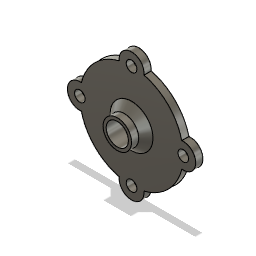
Diode_Holder_Mirror_Mount v5 (Autodesk Fusion 360 design; units mm, degrees)
Autodesk Fusion 360 part; units mm, degrees
note: some values were not read from the file. Set by a fixed rule: which sketch regions a step uses.
sketch "Sketch1" plane through (0, 0, 0) normal (0, 0, 1) x (1, 0, 0)
  circle A0 centre (0, 0) radius 11
  circle A1 centre (0, 0) radius 12.5
  circle A2 centre (0, 0) radius 14.5
  line L0 (0, 0) -> (0, 14.5)
  line L1 (0, 0) -> (14.5, 0)
  line L2 (0, 0) -> (-14.5, 0)
  line L3 (0, 0) -> (0, -14.5)
  circle A3 centre (0, 14.5) radius 3.5
  circle A4 centre (14.5, 0) radius 3.5
  circle A5 centre (0, -14.5) radius 3.5
  circle A6 centre (-14.5, 0) radius 3.5
  circle A7 centre (-14.5, 0) radius 1.5
  circle A8 centre (0, 14.5) radius 1.5
  circle A9 centre (14.5, 0) radius 1.5
  circle A10 centre (0, -14.5) radius 1.5
  dimension "d1" = 22
  dimension "d2" = 25
  dimension "d3" = 29
  dimension "d4" = 7
  dimension "d5" = 3
  dimension "d6" = 3
  dimension "d7" = 3
  dimension "d8" = 3
  constraint coincident A0.centre A1.centre
  constraint coincident A2 L0.end
  constraint vertical L0
  constraint coincident A2 L1.end
  constraint perpendicular L0 L1
  constraint coincident A2 L2.end
  constraint perpendicular L0 L2
  constraint coincident A2 L3.end
  constraint perpendicular L2 L3
  constraint coincident L0.end A3.centre
  constraint coincident L1.end A4.centre
  constraint tangent A0 A4
  constraint coincident L3.end A5.centre
  constraint tangent A0 A5
  constraint coincident L2.end A6.centre
  constraint concentric A6 A7
  constraint concentric A3 A8
  constraint concentric A4 A9
  constraint concentric A5 A10
  measures "d1" diameter of A0
  measures "d2" diameter of A1
  measures "d3" diameter of A2
  measures "d4" diameter of A3
  measures "d5" diameter of A7
  measures "d6" diameter of A8
  measures "d7" diameter of A9
  measures "d8" diameter of A10
extrude "Extrude1" add sketch "Sketch1" along normal blind 1 contours A0 A1 A4 A5 | A1 L1 A4 | A0 A1 A3 A4 | A1 L1 A4 | A1 L0 A3 | A0 A1 A3 A6 | A1 L0 A3 | A0 A1 A5 A6 | A1 L3 A5 | A1 L3 A5 | A1 A2 L1 A4 A9 | A1 A2 L1 A4 A9 | A1 A2 A3 A4 | A1 A2 A4 A5 | A1 L2 A6 | A1 L2 A6 | A1 A2 L0 A3 A8 | A1 A2 L0 A3 A8 | A1 A2 A3 A6 | A1 A2 L3 A5 A10 | A1 A2 L3 A5 A10 | A1 A2 A5 A6 | A2 A4 A9 | A1 A2 L2 A6 A7 | A1 A2 L2 A6 A7 | A2 A3 A8 | A2 A5 A10 | A2 A6 A7
sketch "Sketch2" plane through (0, 0, 1) normal (0, 0, 1) x (1, 0, 0)
  circle A0 centre (0, -14.5) radius 1.5
  circle A1 centre (14.5, 0) radius 1.5
  circle A2 centre (-14.5, 0) radius 1.5
  circle A3 centre (0, 14.5) radius 1.5
  circle A4 centre (0, 0) radius 11
  arc A5 (-3.4744, 14.0776) -> (-14.0776, 3.4744) centre (0, 0) ccw
  arc A6 (-14.0776, 3.4744) -> (-14.0776, -3.4744) centre (-14.5, 0) ccw
  arc A7 (-14.0776, -3.4744) -> (-3.4744, -14.0776) centre (0, 0) ccw
  arc A8 (-3.4744, -14.0776) -> (3.4744, -14.0776) centre (0, -14.5) ccw
  arc A9 (3.4744, -14.0776) -> (14.0776, -3.4744) centre (0, 0) ccw
  arc A10 (14.0776, -3.4744) -> (14.0776, 3.4744) centre (14.5, 0) ccw
  arc A11 (14.0776, 3.4744) -> (3.4744, 14.0776) centre (0, 0) ccw
  arc A12 (3.4744, 14.0776) -> (-3.4744, 14.0776) centre (0, 14.5) ccw
  circle A13 centre (0, 0) radius 11
  circle A14 centre (0, 0) radius 12.375
  circle A15 centre (0, 0) radius 14.5
  circle A16 centre (0, 14.5) radius 3.5
  circle A17 centre (14.5, 0) radius 3.5
  circle A18 centre (0, -14.5) radius 3.5
  circle A19 centre (-14.5, 0) radius 3.5
  dimension "d11" = 24.75
  constraint coincident A4.centre A5.centre
  constraint concentric A3 A16
  constraint concentric A1 A17
  constraint concentric A0 A18
  constraint concentric A2 A19
  measures "d11" diameter of A14
extrude "Extrude2" add sketch "Sketch2" along normal blind 1.25 contours A0 A8 A15 A18 | A0 A14 A15 A18 | A9 A14 A15 A17 A18 | A7 A14 A15 A18 A19 | A1 A10 A15 A17 | A1 A14 A15 A17 | A2 A6 A15 A19 | A2 A14 A15 A19 | A5 A14 A15 A16 A19 | A11 A14 A15 A16 A17 | A3 A12 A15 A16 | A3 A14 A15 A16
extrude "Extrude3" cut 1 faces at (2.5265, 13.3305, 2.25) along direction (0, 0, -1) blind 1.25
sketch "Sketch3" plane through (0, 0, 1) normal (0, 0, 1) x (1, 0, 0)
  arc A0 (-3.4744, 14.0776) -> (-14.0776, 3.4744) centre (0, 0) ccw
  arc A1 (-14.0776, 3.4744) -> (-14.0776, -3.4744) centre (-14.5, 0) ccw
  arc A2 (-14.0776, -3.4744) -> (-3.4744, -14.0776) centre (0, 0) ccw
  arc A3 (-3.4744, -14.0776) -> (3.4744, -14.0776) centre (0, -14.5) ccw
  arc A4 (3.4744, -14.0776) -> (14.0776, -3.4744) centre (0, 0) ccw
  arc A5 (14.0776, -3.4744) -> (14.0776, 3.4744) centre (14.5, 0) ccw
  arc A6 (14.0776, 3.4744) -> (3.4744, 14.0776) centre (0, 0) ccw
  arc A7 (3.4744, 14.0776) -> (-3.4744, 14.0776) centre (0, 14.5) ccw
  circle A8 centre (0, 14.5) radius 1.5
  circle A9 centre (14.5, 0) radius 1.5
  circle A10 centre (-14.5, 0) radius 1.5
  circle A11 centre (0, -14.5) radius 1.5
  circle A12 centre (0, 0) radius 11
  circle A13 centre (0, 0) radius 3.05
  dimension "d16" = 6.1
  constraint coincident A0.centre A2.centre
  measures "d16" diameter of A13
extrude "Extrude4" add sketch "Sketch3" along normal blind 2 contours A0 A1 A2 A3 A4 A5 A6 A7 | A12
sketch "Sketch4" plane through (0, 0, 3) normal (0, 0, 1) x (1, 0, 0)
  circle A0 centre (-14.5, 0) radius 1.5
  circle A1 centre (0, 14.5) radius 1.5
  circle A2 centre (0, 0) radius 3.05
  circle A3 centre (0, -14.5) radius 1.5
  circle A4 centre (14.5, 0) radius 1.5
  arc A5 (3.4744, 14.0776) -> (-3.4744, 14.0776) centre (0, 14.5) ccw
  arc A6 (-3.4744, 14.0776) -> (-14.0776, 3.4744) centre (0, 0) ccw
  arc A7 (-14.0776, 3.4744) -> (-14.0776, -3.4744) centre (-14.5, 0) ccw
  arc A8 (-14.0776, -3.4744) -> (-3.4744, -14.0776) centre (0, 0) ccw
  arc A9 (-3.4744, -14.0776) -> (3.4744, -14.0776) centre (0, -14.5) ccw
  arc A10 (3.4744, -14.0776) -> (14.0776, -3.4744) centre (0, 0) ccw
  arc A11 (14.0776, -3.4744) -> (14.0776, 3.4744) centre (14.5, 0) ccw
  arc A12 (14.0776, 3.4744) -> (3.4744, 14.0776) centre (0, 0) ccw
  circle A13 centre (0, 0) radius 1.5
  dimension "d19" = 3
  constraint coincident A2.centre A6.centre
  measures "d19" diameter of A13
extrude "Extrude5" cut sketch "Sketch4" against normal blind 1 contours A5 A6 A7 A8 A9 A10 A11 A12
sketch "Sketch5" plane through (0, 0, 2) normal (0, 0, 1) x (1, 0, 0)
  circle A0 centre (0, -14.5) radius 1.5
  circle A1 centre (0, 0) radius 3.05
  circle A2 centre (14.5, 0) radius 1.5
  circle A3 centre (0, 14.5) radius 1.5
  circle A4 centre (-14.5, 0) radius 1.5
  arc A5 (14.0776, 3.4744) -> (3.4744, 14.0776) centre (0, 0) ccw
  arc A6 (3.4744, 14.0776) -> (-3.4744, 14.0776) centre (0, 14.5) ccw
  arc A7 (-3.4744, 14.0776) -> (-14.0776, 3.4744) centre (0, 0) ccw
  arc A8 (-14.0776, 3.4744) -> (-14.0776, -3.4744) centre (-14.5, 0) ccw
  arc A9 (-14.0776, -3.4744) -> (-3.4744, -14.0776) centre (0, 0) ccw
  arc A10 (-3.4744, -14.0776) -> (3.4744, -14.0776) centre (0, -14.5) ccw
  arc A11 (3.4744, -14.0776) -> (14.0776, -3.4744) centre (0, 0) ccw
  arc A12 (14.0776, -3.4744) -> (14.0776, 3.4744) centre (14.5, 0) ccw
  circle A13 centre (0, 0) radius 3.05
  circle A14 centre (0, 0) radius 4
  dimension "d22" = 8
  constraint concentric A1 A13
  constraint concentric A1 A14
  measures "d22" diameter of A14
extrude "Extrude6" add sketch "Sketch5" along normal blind 4 contours A14
chamfer "Chamfer1" distance 2 angle 45 1 edges at (-3.7293, 1.4465, 2)
extrude "Extrude7" add 1 faces at (8.2977, -0.698, 1) along direction (0, 0, -1) blind 1
sketch "Sketch7" plane through (0, 0, 6) normal (0, 0, 1) x (1, 0, 0)
  circle A0 centre (0, 0) radius 3.05
  circle A1 centre (0, 0) radius 4
  circle A2 centre (0, 0) radius 3.125
  dimension "d28" = 6.25
  constraint coincident A0.centre A1.centre
  measures "d28" diameter of A2
extrude "Extrude8" cut sketch "Sketch7" against normal blind 100 contours A2
